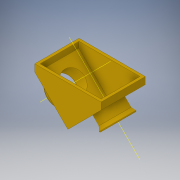
# Autodesk Inventor part: Chamber3-part1
Saved by Autodesk Inventor 2017 (Build 210142000, 142)
## iProperties
Created: 2017-05-09
Part Number: Chamber3-part1
Material: Generic
Document SubType Name: Modeling
Designer: nvladim
Density: 1 g/cm^3
Appearance: Gold
Author: nvladim
Autodesk Inventor part; units mm, degrees
ref_plane "YZ Plane" through (0, 0, 0) normal (1, 0, 0) x (0, 1, 0)
ref_plane "XZ Plane" through (0, 0, 0) normal (0, 1, 0) x (-1, 0, 0)
ref_plane "XY Plane" through (0, 0, 0) normal (0, 0, 1) x (1, 0, 0)
sketch "Sketch1" plane through (0, 0, 0) normal (0, 0, 1) x (1, 0, 0)
  line L0 (0, 0) -> (37.4998, 37.4998)
  line L1 (0, 0) -> (60.1041, 0) construction
  line L2 (-37.4998, 37.4998) -> (0, 0)
  line L3 (-37.5, 45.4552) -> (37.5, 45.4552)
  line L4 (37.5, 45.4552) -> (37.5, 37.4998)
  line L5 (-37.5, 37.4998) -> (-37.5, 45.4552)
  line L6 (0, 40.2877) -> (0, 0)
  line L7 (37.5, 37.4998) -> (37.4998, 37.4998)
  line L8 (-37.4998, 37.4998) -> (-37.5, 37.4998)
  line L9 (-25.0019, 42.5142) -> (24.9981, 42.5142) construction
  line L10 (24.9981, 42.5142) -> (24.9981, 37.5142) construction
  dimension "d0" = 45
  dimension "d39" = 75
  dimension "d41" = 50
  dimension "d42" = 5
  constraints: 22 end point, 3 horizontal, 3 parallel, 2 perpendicular, 2 vertical, 1 other
  measures "d0" angle of L1 L0
  measures "d39" distance of L4.end L5.start
  measures "d41" distance of L9.start L9.end
  measures "d42" distance of L9.end L10.end
extrude "Extrusion1" add sketch "Sketch1" along normal blind 50
shell "Shell2" thickness 3 removed faces 1 at (12.5, 45.4552, 16.6667)
sketch "Sketch2" plane through (37.4998, 37.4998, 50) normal (0.7071068, -0.7071068, 0) x (-0.7071068, -0.7071068, 0)
  circle A0 centre (23.0328, 25) radius 13
  line L0 (53.0328, 0) -> (0, 0) projected
  line L1 (53.0328, 50) -> (53.0328, 0) projected
  circle A1 centre (23.0328, 25) radius 15
  dimension "d5" = 26
  dimension "d6" = 25
  dimension "d7" = 30
  dimension "d26" = 30
  constraints: 2 centre point, 1 coincident
  measures "d5" diameter of A0
  measures "d6" distance from line of L0 A0.centre
  measures "d7" distance from line of L1 A0.centre
  measures "d26" diameter of A1
sketch "Sketch3" plane through (0, 0, 50) normal (-0.7071068, -0.7071068, 0) x (-0.7071068, 0.7071068, 0)
  circle A0 centre (30, 25) radius 13
  line L0 (0, 50) -> (0, 0) projected
  line L1 (53.0328, 0) -> (0, 0) projected
  circle A1 centre (30, 25) radius 15
  dimension "d8" = 26
  dimension "d9" = 30
  dimension "d10" = 25
  dimension "d29" = 30
  constraints: 2 centre point, 1 coincident
  measures "d8" diameter of A0
  measures "d9" distance from line of L0 A0.centre
  measures "d10" distance from line of L1 A0.centre
  measures "d29" diameter of A1
extrude "Extrusion2" cut sketch "Sketch3" against normal through all contours A0
extrude "Extrusion3" cut sketch "Sketch2" against normal blind 10 contours A0
extrude "Extrusion6" add sketch "Sketch2" along normal blind 15
extrude "Extrusion7" add sketch "Sketch3" along normal blind 15
sketch "Sketch9" plane through (-31.8198, 10.6066, 25) normal (-0.7071068, -0.7071068, 0) x (-0.7071068, 0.7071068, 0)
  circle A0 centre (0, 0) radius 15
  circle A1 centre (0, 0) radius 17
  point P0 (-30, 25)
  dimension "d81" = 34
  constraints: 2 centre point, 1 coincident
  measures "d81" diameter of A1
extrude "Extrusion12" add sketch "Sketch9" against normal blind 5
chamfer "Chamfer2" distance 4 angle 25 1 edges at (-16.2635, 2.1213, 25) measured on face at (-41.4446, 24.9455, 26.3679)
fillet "Fillet3" radius 3 1 edges at (-22.6274, 1.4142, 25)
fillet "Fillet4" radius 0.5 1 edges at (-19.799, -1.4142, 25)
sketch "Sketch16" plane through (31.8198, 10.6066, 25) normal (0.7071068, -0.7071068, 0) x (-0.7071068, -0.7071068, 0)
  circle A0 centre (0, 0) radius 17
  circle A1 centre (0, 0) radius 13 projected
  point P0 (30, 25)
  dimension "d134" = 34
  constraints: 1 centre point
  measures "d134" diameter of A0
extrude "Extrusion19" add sketch "Sketch16" against normal blind 5
chamfer "Chamfer3" distance 2 distance2 4 1 edges at (40.3051, 26.163, 25) measured on face at (16.954, 2.8119, 27.5527)
fillet "Fillet7" radius 3 1 edges at (41.0122, 19.799, 25)
fillet "Fillet8" radius 0.5 1 edges at (43.8406, 22.6274, 25)
body "Solid1"
